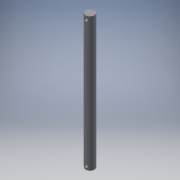
# Autodesk Inventor part: Cylindar
Saved by Autodesk Inventor 2018 (Build 220112000, 112)
## iProperties
Created: 2018-01-12
Part Number: Cylindar
Material: Generic
Document SubType Name: Modeling
Designer: Apple
Density: 1 g/cm^3
Appearance: Default
Author: Apple
Autodesk Inventor part; units mm, degrees
ref_plane "YZ Plane" through (0, 0, 0) normal (1, 0, 0) x (0, 1, 0)
ref_plane "XZ Plane" through (0, 0, 0) normal (0, 1, 0) x (-1, 0, 0)
ref_plane "XY Plane" through (0, 0, 0) normal (0, 0, 1) x (1, 0, 0)
sketch "Sketch1" plane through (0, 0, 0) normal (0, 1, 0) x (-1, 0, 0)
  circle A0 centre (0, 0) radius 15.875
  dimension "d0" = 31.75
  constraints: 1 centre point, 1 coincident
  measures "d0" diameter of A0
extrude "Extrusion1" add sketch "Sketch1" along normal blind 482.6
sketch "Sketch2" plane through (0, 0, 0) normal (0, 0, 1) x (1, 0, 0)
  circle A0 centre (0, 12.7) radius 6.35
  line L0 (-15.875, 0) -> (15.875, 0) projected
  circle A1 centre (0, 469.9) radius 6.35
  line L1 (15.875, 482.6) -> (-15.875, 482.6) projected
  point P0 (0, 0)
  dimension "d3" = 12.7
  dimension "d6" = 12.7
  dimension "d7" = 12.7
  dimension "d8" = 12.7
  constraints: 2 centre point
  measures "d3" diameter of A0
  measures "d6" distance from line of A0.centre L0
  measures "d7" diameter of A1
  measures "d8" distance from line of A1.centre L1
extrude "Extrusion2" cut sketch "Sketch2" along normal mid plane 50.8
equation "\"d8\" = d6"
body "Solid1"
